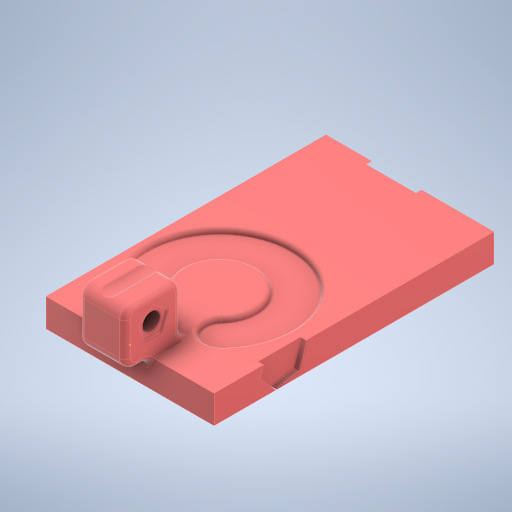
# Autodesk Inventor part: 零件4
Saved by Autodesk Inventor 2023 (Build 270158000, 158)
## iProperties
Created: 2023-09-13
Part Number: 零件4
Material: 常规
Document SubType Name: Modeling
Designer: Administrator
Density: 1 g/cm^3
Appearance: 平滑 - 红色
Author: Administrator
Autodesk Inventor part; units mm, degrees
ref_plane "YZ Plane" through (0, 0, 0) normal (1, 0, 0) x (0, 1, 0)
ref_plane "XZ Plane" through (0, 0, 0) normal (0, 1, 0) x (-1, 0, 0)
ref_plane "XY Plane" through (0, 0, 0) normal (0, 0, 1) x (1, 0, 0)
sketch "草图1" plane through (0, 0, 0) normal (0, 1, 0) x (-1, 0, 0)
  line L0 (0, 0) -> (15, 0)
  line L1 (15, 0) -> (15, -50)
  line L2 (15, -50) -> (0, -50)
  line L3 (0, -50) -> (0, 0)
  dimension "d0" = 50
  dimension "d1" = 15
  constraints: 8 end point, 2 parallel, 1 horizontal, 1 perpendicular
  measures "d0" distance of L0.end L1.end
  measures "d1" distance of L1.end L2.end
extrude "拉伸1" add sketch "草图1" along normal blind 5
sketch "草图2" plane through (0, 0, 0) normal (1, 0, 0) x (0, 1, 0)
  point P0 (0, 0)
sketch "草图3" plane through (0, 0, 0) normal (1, 0, 0) x (0, 1, 0)
  line L0 (15, 5) -> (5, 5)
  line L1 (5, 5) -> (5, -5)
  line L2 (5, -5) -> (15, -5)
  line L3 (15, -5) -> (15, 5)
  line L4 (0, 0) -> (5, 0) projected
  line L5 (5, 0) -> (5, -50) projected
  dimension "d4" = 10
  dimension "d5" = 10
  dimension "d6" = 5
  dimension "d7" = 10
  constraints: 8 end point, 2 parallel, 1 horizontal, 1 perpendicular
  measures "d4" distance of L2.end L0.start
  measures "d5" distance of L1.end L2.end
  measures "d6" distance between parallel lines of L4 L0
  measures "d7" distance between parallel lines of L5 L3
extrude "拉伸2" add sketch "草图3" against normal blind 4.125
mirror "镜像1" about plane through (0, 0, 0) normal (1, 0, 0)
sketch "草图4" plane through (0, 0, 0) normal (1, 0, 0) x (0, 1, 0)
  circle A0 centre (10.5, 0) radius 1.6
  line L0 (5, -50) -> (5, 0) projected
  line L1 (0, 0) -> (5, 0) projected
  line L2 (15, 5) -> (15, -5) projected
  dimension "d10" = 3.2
  dimension "d12" = 0
  dimension "d22" = 4.5
  constraints: 1 centre point
  measures "d10" diameter of A0
  measures "d12" distance from line of L1 A0.centre
  measures "d22" distance from line of A0.centre L2
extrude "拉伸3" cut sketch "草图4" along normal mid plane 10
fillet "圆角1" radius 2 3 edges at (0, 5, 0) (0, 5, 5) (0, 15, 5)
fillet "圆角2" radius 2 2 edges at (0, 15, -5) (0, 5, -5)
sketch "草图5" plane through (0, 0, 0) normal (0, 1, 0) x (-1, 0, 0)
  point P0 (0, 0)
sketch "草图6" plane through (0, 0, 0) normal (0, 0, 1) x (1, 0, 0)
  circle A0 centre (-0.125, 16.5) radius 2
  line L0 (4.125, 15) -> (-4.125, 15) projected
  line L1 (-4.125, 7) -> (-4.125, 13) projected
  point P0 (0, 0)
  dimension "d17" = 4
  dimension "d18" = 1.5
  dimension "d19" = 4
  constraints: 1 centre point
  measures "d17" diameter of A0
  measures "d18" distance from line of L0 A0.centre
  measures "d19" distance from line of L1 A0.centre
extrude "拉伸4" cut sketch "草图6" along normal mid plane 10
fillet "圆角3" radius 1 18 edges at (4.125, 15, 0) (4.125, 14.4142, -4.4142) (4.125, 10, -5) (4.125, 5.5858, -5.5858) (4.125, 10, 5) (4.125, 5.5858, 4.4142) (4.125, 5, 2.5) (4.125, 4.4142, 0.5858) (4.125, 14.4142, 4.4142) (-4.125, 10, 5) (-4.125, 5.5858, 4.4142) (-4.125, 5, 2.5) (-4.125, 4.4142, 0.5858) (-4.125, 15, 0) (-4.125, 14.4142, -4.4142) (-4.125, 10, -5) (-4.125, 5.5858, -5.5858) (-4.125, 14.4142, 4.4142)
sketch "草图7" plane through (0, 5, 0) normal (0, 1, 0) x (1, 0, 0)
  arc A0 (6.1366, 10.4655) -> (-8.2833, 10.5134) centre (-1.0516, 17.0329) ccw construction
  arc A1 (8.3868, 8.4097) -> (-10.5472, 8.4726) centre (-1.0516, 17.0329) ccw
  arc A2 (3.8864, 12.5214) -> (-6.0195, 12.5543) centre (-1.0516, 17.0329) ccw
  arc A3 (3.8864, 12.5214) -> (8.3868, 8.4097) centre (6.1366, 10.4655) ccw
  arc A4 (-10.5472, 8.4726) -> (-6.0195, 12.5543) centre (-8.2833, 10.5134) ccw
  arc A5 (4.0807, 21.859) -> (-6.0195, 33.0511) centre (-0.9036, 27.5144) ccw construction
  arc A6 (5.2592, 20.5219) -> (-7.2291, 34.3602) centre (-0.9036, 27.5144) ccw
  arc A7 (2.9023, 23.1961) -> (-4.8099, 31.7421) centre (-0.9036, 27.5144) ccw
  arc A8 (2.9023, 23.1961) -> (5.2592, 20.5219) centre (4.0807, 21.859) ccw
  arc A9 (-7.2291, 34.3602) -> (-4.8099, 31.7421) centre (-6.0195, 33.0511) ccw
  arc A10 (-7.2291, 34.3602) -> (-0.9036, 40.3394) centre (3.2207, 29.6408) ccw construction
  arc A11 (-7.2627, 34.3754) -> (-0.9169, 40.3739) centre (3.2207, 29.6408) ccw
  arc A12 (-7.1954, 34.345) -> (-0.8904, 40.305) centre (3.2207, 29.6408) ccw
  arc A13 (-7.1954, 34.345) -> (-7.2627, 34.3754) centre (-7.2291, 34.3602) ccw
  arc A14 (-0.9169, 40.3739) -> (-0.8904, 40.305) centre (-0.9036, 40.3394) ccw
  point P0 (0, 0)
  constraints: 30 point on circle, 15 centre point, 12 tangent
extrude "拉伸5" cut sketch "草图7" against normal blind 1 contours A3 A2 A11 A1 | A11 A2 A12 A1 | A12 A2 A8 A6 A1 | A6 A8 A2 A7 A1 | A11 A1 A12 A2 | A2 A4 A1 A11 | A7 A8 A2 A12 A1
fillet "圆角4" radius 1 4 edges at (4.0807, 5, -8.2153) (-1.0294, 5, -23.7214) (-6.2425, 5, -8.2496) (-1.0092, 5, -29.8173)
sketch "草图8" plane through (0, 5, 0) normal (0, 1, 0) x (1, 0, 0)
  point P0 (0, 0)
sketch "草图9" plane through (0, 0, -50) normal (0, 0, 1) x (1, 0, 0)
  arc A0 (3.8532, 1.8896) -> (-8.818, 1.6673) centre (-2.3802, -4.0474) ccw construction
  arc A1 (4.9239, 2.9094) -> (-9.9238, 2.6489) centre (-2.3802, -4.0474) ccw
  arc A2 (2.7826, 0.8698) -> (-7.7122, 0.6857) centre (-2.3802, -4.0474) ccw
  arc A3 (2.7826, 0.8698) -> (4.9239, 2.9094) centre (3.8532, 1.8896) ccw
  arc A4 (-9.9238, 2.6489) -> (-7.7122, 0.6857) centre (-8.818, 1.6673) ccw
  point P0 (0, 0)
  constraints: 10 point on circle, 5 centre point, 4 tangent
extrude "拉伸6" cut sketch "草图9" along normal blind 1
sketch "草图10" plane through (15, 0, 0) normal (1, 0, 0) x (0, 0, -1)
  line L0 (8.4097, 4) -> (29.8174, 4) projected
  line L1 (15.2277, 0.8151) -> (11.0616, -0.031)
  line L2 (11.0616, -0.031) -> (8.2458, 3.1539)
  line L3 (8.2458, 3.1539) -> (9.5961, 7.1849)
  line L4 (9.5961, 7.1849) -> (13.7622, 8.031)
  line L5 (13.7622, 8.031) -> (16.578, 4.8461)
  line L6 (16.578, 4.8461) -> (15.2277, 0.8151)
  point P0 (0, 0)
  point P1 (12.4119, 4)
  point P2 (8.4726, 4)
  constraints: 12 end point, 1 point on line, 13 other
extrude "拉伸7" cut sketch "草图10" against normal blind 1
sketch "草图11" plane through (-15, 0, -50) normal (-1, 0, 0) x (0, 0, 1)
  line L0 (5.5098, 1.69) -> (3.9929, 0.1998)
  line L1 (3.9929, 0.1998) -> (2.1069, 1.182)
  line L2 (2.1069, 1.182) -> (2.4582, 3.2792)
  line L3 (2.4582, 3.2792) -> (4.5613, 3.5932)
  line L4 (4.5613, 3.5932) -> (5.5098, 1.69)
  point P0 (50, 0)
  point P1 (3.7258, 1.9889)
  constraints: 10 end point, 11 other
extrude "拉伸8" cut sketch "草图11" against normal blind 1
sketch "草图12" plane through (-4.125, 0, 0) normal (-1, 0, 0) x (0, 0, 1)
  line L0 (1.3276, 7.7307) -> (-2.1715, 8.3439)
  line L1 (-2.1715, 8.3439) -> (-2.6696, 11.8612)
  line L2 (-2.6696, 11.8612) -> (0.5216, 13.4218)
  line L3 (0.5216, 13.4218) -> (2.992, 10.8691)
  line L4 (2.992, 10.8691) -> (1.3276, 7.7307)
  point P0 (0, 0)
  point P1 (0, 10.4453)
  constraints: 10 end point, 11 other
extrude "拉伸9" cut sketch "草图12" against normal blind 0.3
sketch "草图13" plane through (4.125, 7, -4) normal (1, 0, 0) x (0, 0, -1)
  circle A0 centre (-4, 3.5) radius 1.6 projected
  line L0 (-5.3276, 0.7307) -> (-1.8285, 1.3439) projected
  line L1 (-2.5195, 1.2228) -> (-5.7082, 1.3882)
  line L2 (-5.7082, 1.3882) -> (-6.5363, 4.472)
  line L3 (-6.5363, 4.472) -> (-3.8593, 6.2125)
  line L4 (-3.8593, 6.2125) -> (-1.3768, 4.2044)
  line L5 (-1.3768, 4.2044) -> (-2.5195, 1.2228)
  point P0 (-4, -7)
  constraints: 10 end point, 1 coincident, 1 point on line, 11 other
extrude "拉伸10" cut sketch "草图13" against normal blind 0.3 contours A0 | L1 L2 L3 L4 L5
